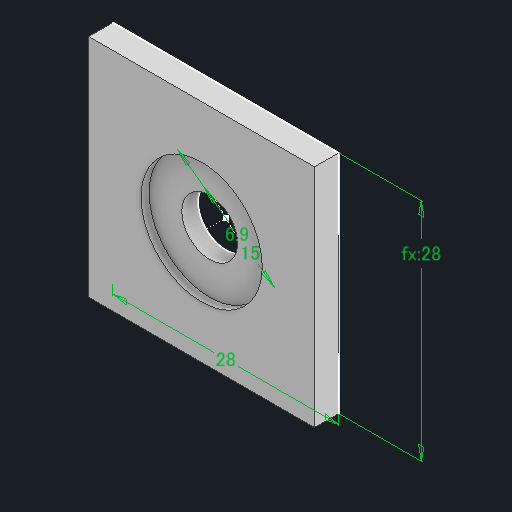
# Autodesk Inventor part: baicPart
Saved by Autodesk Inventor 2025.2 (Build 292293000, 293)
## iProperties
Company: FC-TORQUE
Created: 2025-03-14
Part Number: baicPart
Material: 一般
Document SubType Name: Modeling
Designer: Keito Tamura
Density: 1 g/cm^3
Appearance: 既定
Author: Keito Tamura
Autodesk Inventor part; units mm, degrees
ref_plane "YZ Plane" through (0, 0, 0) normal (1, 0, 0) x (0, 1, 0)
ref_plane "XZ Plane" through (0, 0, 0) normal (0, 1, 0) x (-1, 0, 0)
ref_plane "XY Plane" through (0, 0, 0) normal (0, 0, 1) x (1, 0, 0)
sketch "スケッチ1" plane through (0, 0, 0) normal (0, 0, 1) x (1, 0, 0)
  circle A0 centre (0, 0) radius 3.45
  circle A1 centre (0, 0) radius 7.5
  line L0 (-14, 14) -> (14, 14)
  line L1 (14, 14) -> (14, -14)
  line L2 (14, -14) -> (-14, -14)
  line L3 (-14, -14) -> (-14, 14)
  line L4 (-14, 14) -> (14, -14) construction
  line L5 (14, 14) -> (-14, -14) construction
  dimension "d0" = 6.9
  dimension "d1" = 15
  dimension "d2" = 28
  dimension "d3" = 28
  constraints: 12 end point, 2 centre point, 2 coincident, 2 midpoint, 2 parallel, 1 horizontal, 1 perpendicular
  measures "d0" diameter of A0
  measures "d1" diameter of A1
  measures "d2" distance of L1.end L2.end
  measures "d3" distance of L0.end L1.end
extrude "押し出し1" add sketch "スケッチ1" along normal blind 3 contours L0 L1 L2 L3
extrude "押し出し2" add sketch "スケッチ1" along normal blind 2 contours A1
equation "\"d3\" = d2"
